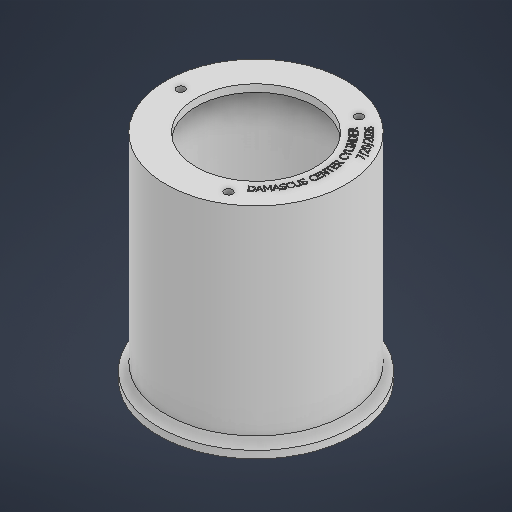
# Autodesk Inventor part: Mithril Center Cylinder
Saved by Autodesk Inventor 2026.3 (Build 303398000, 398)
## iProperties
Created: 2026-03-06
Part Number: Mithril Center Cylinder
Material: Generic
Document SubType Name: Modeling
Designer: mumin
Density: 1 g/cm^3
Appearance: Default
Author: mumin
Autodesk Inventor part; units mm, degrees
note: some values were not read from the file. Chosen so that the rebuilt part matches the saved one: direction of "Hole1".
ref_plane "YZ Plane" through (0, 0, 0) normal (1, 0, 0) x (0, 1, 0)
ref_plane "XZ Plane" through (0, 0, 0) normal (0, 1, 0) x (-1, 0, 0)
ref_plane "XY Plane" through (0, 0, 0) normal (0, 0, 1) x (1, 0, 0)
sketch "Sketch1" plane through (0, 0, 0) normal (1, 0, 0) x (0, 1, 0)
  line L0 (0, 0) -> (100, 0)
  line L1 (145, -40.5) -> (140, -40.5)
  line L2 (140, -40.5) -> (140, -56)
  line L3 (140, -56) -> (0, -56)
  line L4 (0, -56) -> (0, -66)
  line L5 (0, -66) -> (5, -66)
  line L6 (5, -66) -> (5, -61)
  line L7 (5, -61) -> (145, -61)
  line L8 (145, -61) -> (145, -40.5)
  line L9 (5, -66) -> (9.9531, -61)
  point P0 (142.5, -40.5)
  dimension "d0" = 100
  dimension "d1" = 81
  dimension "d2" = 122
  dimension "d3" = 145
  dimension "d4" = 5
  dimension "d5" = 5
  dimension "d6" = 5
  dimension "d7" = 10
  constraints: 20 end point, 7 perpendicular, 2 horizontal, 2 point on line, 1 midpoint
  measures "d0" distance of L0.start L0.end
  measures "d1" diameter of point (142.5, -40.5) L0
  measures "d2" diameter of L7 L0
  measures "d3" distance between parallel lines of L4 L8
  measures "d4" distance between parallel lines of L2 L8
  measures "d5" distance between parallel lines of L4 L6
  measures "d6" distance between parallel lines of L7 L3
  measures "d7" distance between parallel lines of L5 L3
revolve "Revolution1" add sketch "Sketch1" angle 360 about axis through (0, 0, 0) along (0, 1, 0)
sketch "Sketch2" plane through (0, 145, 0) normal (0, 1, 0) x (1, 0, 0)
  circle A0 centre (0, 0) radius 51
  point P0 (-51, 0)
  point P1 (25.5, -44.1673)
  point P2 (25.5, 44.1673)
  dimension "d9" = 102
  dimension "d12" = 360
  constraints: 1 coincident, 1 horizontal alignment, 6 other
hole "Hole1" at (-51, 145, 0) at (25.5, 145, 44.1673) at (25.5, 145, -44.1673) direction (0, -1, 0) diameter 5.5 end up to surface
sketch "Sketch3" plane through (0, 145, 0) normal (0, 1, 0) x (1, 0, 0)
  circle A0 centre (25.5, 44.1673) radius 2.75 projected
  circle A1 centre (25.5, -44.1673) radius 2.75 projected
  circle A2 centre (-51, 0) radius 2.75 projected
  circle A3 centre (0, 0) radius 40.5 projected
  circle A4 centre (0, 0) radius 61 projected
  spline S0 degree 2 poles (32.8898, -33.2836) (33.3048, -33.7392) (33.6033, -34.8089) (33.4798, -35.2962) knots 0 0 0 1 2 2 2
  spline S1 degree 2 poles (33.4798, -35.2962) (33.3713, -35.6861) (32.9491, -36.2679) (32.5447, -36.6362) knots 0 0 0 1 2 2 2
  line L0 (32.5447, -36.6362) -> (31.779, -37.3335)
  line L1 (31.779, -37.3335) -> (28.749, -34.0065)
  line L2 (28.749, -34.0065) -> (29.5066, -33.3165)
  spline S2 degree 2 poles (29.5066, -33.3165) (29.9757, -32.8893) (30.6373, -32.5433) (30.9389, -32.4954) knots 0 0 0 1 2 2 2
  spline S3 degree 2 poles (30.9389, -32.4954) (31.4537, -32.4162) (32.4478, -32.7983) (32.8898, -33.2836) knots 0 0 0 1 2 2 2
  spline S4 degree 2 poles (32.4238, -33.6981) (32.0752, -33.3152) (31.3282, -33.0041) (30.9375, -33.0788) knots 0 0 0 1 2 2 2
  spline S5 degree 2 poles (30.9375, -33.0788) (30.6638, -33.1357) (30.1761, -33.4072) (29.8769, -33.6797) knots 0 0 0 1 2 2 2
  line L3 (29.8769, -33.6797) -> (29.5398, -33.9867)
  line L4 (29.5398, -33.9867) -> (31.8725, -36.548)
  line L5 (31.8725, -36.548) -> (32.2095, -36.241)
  spline S6 degree 2 poles (32.2095, -36.241) (32.5034, -35.9734) (32.8623, -35.4739) (32.9276, -35.1827) knots 0 0 0 1 2 2 2
  spline S7 degree 2 poles (32.9276, -35.1827) (33.017, -34.8151) (32.7774, -34.0863) (32.4238, -33.6981) knots 0 0 0 1 2 2 2
  line L6 (34.5192, -34.8294) -> (32.2641, -30.6502)
  line L7 (32.2641, -30.6502) -> (32.7667, -30.1116)
  line L8 (32.7667, -30.1116) -> (37.0917, -32.0726)
  line L9 (37.0917, -32.0726) -> (36.6613, -32.5338)
  line L10 (36.6613, -32.5338) -> (35.4628, -31.9741)
  line L11 (35.4628, -31.9741) -> (34.291, -33.2299)
  line L12 (34.291, -33.2299) -> (34.9322, -34.3868)
  line L13 (34.9322, -34.3868) -> (34.5192, -34.8294)
  line L14 (34.9776, -31.7458) -> (32.9534, -30.8095)
  line L15 (32.9534, -30.8095) -> (34.0297, -32.7616)
  line L16 (34.0297, -32.7616) -> (34.9776, -31.7458)
  line L17 (39.7858, -28.6673) -> (39.4173, -29.1384)
  line L18 (39.4173, -29.1384) -> (36.3639, -26.7503)
  line L19 (36.3639, -26.7503) -> (37.7173, -29.2995)
  line L20 (37.7173, -29.2995) -> (37.4926, -29.5867)
  line L21 (37.4926, -29.5867) -> (34.6992, -28.8788)
  line L22 (34.6992, -28.8788) -> (37.7526, -31.2669)
  line L23 (37.7526, -31.2669) -> (37.4089, -31.7064)
  line L24 (37.4089, -31.7064) -> (33.8643, -28.9341)
  line L25 (33.8643, -28.9341) -> (34.3675, -28.2907)
  line L26 (34.3675, -28.2907) -> (37.0328, -28.9493)
  line L27 (37.0328, -28.9493) -> (35.7289, -26.55)
  line L28 (35.7289, -26.55) -> (36.2411, -25.895)
  line L29 (36.2411, -25.895) -> (39.7858, -28.6673)
  line L30 (40.0329, -28.3201) -> (37.0877, -24.595)
  line L31 (37.0877, -24.595) -> (37.4893, -23.9775)
  line L32 (37.4893, -23.9775) -> (42.0887, -25.1592)
  line L33 (42.0887, -25.1592) -> (41.7448, -25.688)
  line L34 (41.7448, -25.688) -> (40.4674, -25.3445)
  line L35 (40.4674, -25.3445) -> (39.531, -26.7844)
  line L36 (39.531, -26.7844) -> (40.363, -27.8127)
  line L37 (40.363, -27.8127) -> (40.0329, -28.3201)
  line L38 (39.95, -25.2037) -> (37.7941, -24.6325)
  line L39 (37.7941, -24.6325) -> (39.1925, -26.3684)
  line L40 (39.1925, -26.3684) -> (39.95, -25.2037)
  spline S8 degree 2 poles (42.9943, -23.6719) (42.7587, -24.1) (42.2493, -24.6022) (41.9756, -24.7971) knots 0 0 0 1 2 2 2
  line L41 (41.9756, -24.7971) -> (41.3174, -24.435)
  line L42 (41.3174, -24.435) -> (41.3385, -24.3966)
  spline S9 degree 2 poles (41.3385, -24.3966) (41.7237, -24.2714) (42.3525, -23.7641) (42.5195, -23.4606) knots 0 0 0 1 2 2 2
  spline S10 degree 2 poles (42.5195, -23.4606) (42.7586, -23.0261) (42.6419, -22.3834) (42.3448, -22.2199) knots 0 0 0 1 2 2 2
  spline S11 degree 2 poles (42.3448, -22.2199) (42.1084, -22.0898) (41.6861, -22.1613) (41.4737, -22.3732) knots 0 0 0 1 2 2 2
  spline S12 degree 2 poles (41.4737, -22.3732) (41.3224, -22.5272) (41.0851, -22.7921) (40.9028, -22.9873) knots 0 0 0 1 2 2 2
  spline S13 degree 2 poles (40.9028, -22.9873) (40.736, -23.1618) (40.3955, -23.3949) (40.1959, -23.4474) knots 0 0 0 1 2 2 2
  spline S14 degree 2 poles (40.1959, -23.4474) (39.9981, -23.4967) (39.5728, -23.4375) (39.3428, -23.311) knots 0 0 0 1 2 2 2
  spline S15 degree 2 poles (39.3428, -23.311) (38.8636, -23.0473) (38.6264, -21.9428) (38.9446, -21.3645) knots 0 0 0 1 2 2 2
  spline S16 degree 2 poles (38.9446, -21.3645) (39.1274, -21.0322) (39.5819, -20.5164) (39.8453, -20.3326) knots 0 0 0 1 2 2 2
  line L43 (39.8453, -20.3326) -> (40.4715, -20.6771)
  line L44 (40.4715, -20.6771) -> (40.4504, -20.7155)
  spline S17 degree 2 poles (40.4504, -20.7155) (40.1742, -20.8091) (39.5951, -21.2563) (39.4176, -21.579) knots 0 0 0 1 2 2 2
  spline S18 degree 2 poles (39.4176, -21.579) (39.2172, -21.9432) (39.3111, -22.5818) (39.5891, -22.7347) knots 0 0 0 1 2 2 2
  spline S19 degree 2 poles (39.5891, -22.7347) (39.8383, -22.8719) (40.2814, -22.7702) (40.4856, -22.5579) knots 0 0 0 1 2 2 2
  spline S20 degree 2 poles (40.4856, -22.5579) (40.6217, -22.4164) (41.0022, -21.9972) (41.138, -21.8638) knots 0 0 0 1 2 2 2
  spline S21 degree 2 poles (41.138, -21.8638) (41.4859, -21.5266) (42.1949, -21.4256) (42.5624, -21.6278) knots 0 0 0 1 2 2 2
  spline S22 degree 2 poles (42.5624, -21.6278) (42.7956, -21.7561) (43.1392, -22.1908) (43.2025, -22.4462) knots 0 0 0 1 2 2 2
  spline S23 degree 2 poles (43.2025, -22.4462) (43.2713, -22.7297) (43.1929, -23.3109) (42.9943, -23.6719) knots 0 0 0 1 2 2 2
  spline S24 degree 2 poles (44.7609, -20.1361) (44.5784, -20.5338) (44.0014, -21.0836) (43.6204, -21.2058) knots 0 0 0 1 2 2 2
  spline S25 degree 2 poles (43.6204, -21.2058) (43.2427, -21.3294) (42.324, -21.2331) (41.8069, -20.996) knots 0 0 0 1 2 2 2
  spline S26 degree 2 poles (41.8069, -20.996) (41.2932, -20.7603) (40.6509, -20.1488) (40.4831, -19.771) knots 0 0 0 1 2 2 2
  spline S27 degree 2 poles (40.4831, -19.771) (40.3205, -19.3996) (40.3392, -18.5977) (40.5292, -18.1834) knots 0 0 0 1 2 2 2
  spline S28 degree 2 poles (40.5292, -18.1834) (40.6234, -17.9779) (40.8488, -17.6439) (40.9651, -17.5127) knots 0 0 0 1 2 2 2
  spline S29 degree 2 poles (40.9651, -17.5127) (41.069, -17.3999) (41.3178, -17.181) (41.4531, -17.0786) knots 0 0 0 1 2 2 2
  line L45 (41.4531, -17.0786) -> (42.1094, -17.3796)
  line L46 (42.1094, -17.3796) -> (42.0896, -17.4227)
  spline S30 degree 2 poles (42.0896, -17.4227) (41.9899, -17.4652) (41.7009, -17.6054) (41.5369, -17.7268) knots 0 0 0 1 2 2 2
  spline S31 degree 2 poles (41.5369, -17.7268) (41.3793, -17.8431) (41.1012, -18.1609) (40.9917, -18.3995) knots 0 0 0 1 2 2 2
  spline S32 degree 2 poles (40.9917, -18.3995) (40.8716, -18.6614) (40.8728, -19.2276) (40.9977, -19.4975) knots 0 0 0 1 2 2 2
  spline S33 degree 2 poles (40.9977, -19.4975) (41.1275, -19.7656) (41.6724, -20.2482) (42.0669, -20.4291) knots 0 0 0 1 2 2 2
  spline S34 degree 2 poles (42.0669, -20.4291) (42.4879, -20.6222) (43.1872, -20.6982) (43.4766, -20.6183) knots 0 0 0 1 2 2 2
  spline S35 degree 2 poles (43.4766, -20.6183) (43.7578, -20.5386) (44.1746, -20.1721) (44.2932, -19.9136) knots 0 0 0 1 2 2 2
  spline S36 degree 2 poles (44.2932, -19.9136) (44.4011, -19.6782) (44.4691, -19.2239) (44.4543, -19.0286) knots 0 0 0 1 2 2 2
  spline S37 degree 2 poles (44.4543, -19.0286) (44.4365, -18.8399) (44.3594, -18.5358) (44.3253, -18.4439) knots 0 0 0 1 2 2 2
  line L47 (44.3253, -18.4439) -> (44.3435, -18.4041)
  line L48 (44.3435, -18.4041) -> (44.9932, -18.7021)
  spline S38 degree 2 poles (44.9932, -18.7021) (44.9939, -18.8669) (45.0004, -19.1587) (44.976, -19.3521) knots 0 0 0 1 2 2 2
  spline S39 degree 2 poles (44.976, -19.3521) (44.9535, -19.5585) (44.8733, -19.8908) (44.7609, -20.1361) knots 0 0 0 1 2 2 2
  spline S40 degree 2 poles (46.1061, -16.868) (45.9695, -17.2413) (45.5714, -17.7247) (45.3048, -17.8485) knots 0 0 0 1 2 2 2
  spline S41 degree 2 poles (45.3048, -17.8485) (45.0041, -17.9909) (44.3213, -17.9469) (43.8692, -17.7815) knots 0 0 0 1 2 2 2
  line L49 (43.8692, -17.7815) -> (41.2322, -16.8169)
  line L50 (41.2322, -16.8169) -> (41.4377, -16.2552)
  line L51 (41.4377, -16.2552) -> (44.0747, -17.2199)
  spline S42 degree 2 poles (44.0747, -17.2199) (44.3692, -17.3276) (44.7941, -17.3976) (44.9938, -17.3503) knots 0 0 0 1 2 2 2
  spline S43 degree 2 poles (44.9938, -17.3503) (45.2064, -17.2999) (45.5239, -16.9734) (45.6266, -16.6926) knots 0 0 0 1 2 2 2
  spline S44 degree 2 poles (45.6266, -16.6926) (45.7231, -16.4289) (45.6988, -15.954) (45.5689, -15.7784) knots 0 0 0 1 2 2 2
  spline S45 degree 2 poles (45.5689, -15.7784) (45.4468, -15.6133) (45.0805, -15.3939) (44.7962, -15.2899) knots 0 0 0 1 2 2 2
  line L52 (44.7962, -15.2899) -> (42.1455, -14.3202)
  line L53 (42.1455, -14.3202) -> (42.3509, -13.7586)
  line L54 (42.3509, -13.7586) -> (44.988, -14.7232)
  spline S46 degree 2 poles (44.988, -14.7232) (45.4298, -14.8849) (45.9948, -15.2935) (46.1278, -15.5984) knots 0 0 0 1 2 2 2
  spline S47 degree 2 poles (46.1278, -15.5984) (46.2526, -15.8731) (46.2489, -16.4776) (46.1061, -16.868) knots 0 0 0 1 2 2 2
  spline S48 degree 2 poles (47.2439, -13.2996) (47.1117, -13.77) (46.7295, -14.3746) (46.5071, -14.6265) knots 0 0 0 1 2 2 2
  line L55 (46.5071, -14.6265) -> (45.7839, -14.4232)
  line L56 (45.7839, -14.4232) -> (45.7958, -14.381)
  spline S49 degree 2 poles (45.7958, -14.381) (46.1426, -14.1717) (46.6398, -13.535) (46.7336, -13.2015) knots 0 0 0 1 2 2 2
  spline S50 degree 2 poles (46.7336, -13.2015) (46.8679, -12.7241) (46.6084, -12.1245) (46.2819, -12.0327) knots 0 0 0 1 2 2 2
  spline S51 degree 2 poles (46.2819, -12.0327) (46.0222, -11.9597) (45.6271, -12.1251) (45.4684, -12.3797) knots 0 0 0 1 2 2 2
  spline S52 degree 2 poles (45.4684, -12.3797) (45.356, -12.564) (45.1849, -12.8758) (45.0517, -13.1073) knots 0 0 0 1 2 2 2
  spline S53 degree 2 poles (45.0517, -13.1073) (44.9288, -13.3152) (44.65, -13.6194) (44.4676, -13.7158) knots 0 0 0 1 2 2 2
  spline S54 degree 2 poles (44.4676, -13.7158) (44.2862, -13.8087) (43.8585, -13.8476) (43.6058, -13.7765) knots 0 0 0 1 2 2 2
  spline S55 degree 2 poles (43.6058, -13.7765) (43.0792, -13.6284) (42.5976, -12.6065) (42.7763, -11.9711) knots 0 0 0 1 2 2 2
  spline S56 degree 2 poles (42.7763, -11.9711) (42.879, -11.6061) (43.2045, -11.0006) (43.4195, -10.7618) knots 0 0 0 1 2 2 2
  line L57 (43.4195, -10.7618) -> (44.1075, -10.9553)
  line L58 (44.1075, -10.9553) -> (44.0957, -10.9974)
  spline S57 degree 2 poles (44.0957, -10.9974) (43.8478, -11.1512) (43.3854, -11.7182) (43.2856, -12.0727) knots 0 0 0 1 2 2 2
  spline S58 degree 2 poles (43.2856, -12.0727) (43.1731, -12.4729) (43.4095, -13.0735) (43.7149, -13.1594) knots 0 0 0 1 2 2 2
  spline S59 degree 2 poles (43.7149, -13.1594) (43.9887, -13.2364) (44.3972, -13.0369) (44.5479, -12.7838) knots 0 0 0 1 2 2 2
  spline S60 degree 2 poles (44.5479, -12.7838) (44.6484, -12.6151) (44.9238, -12.1205) (45.0258, -11.9598) knots 0 0 0 1 2 2 2
  spline S61 degree 2 poles (45.0258, -11.9598) (45.2881, -11.5525) (45.9558, -11.2932) (46.3595, -11.4068) knots 0 0 0 1 2 2 2
  spline S62 degree 2 poles (46.3595, -11.4068) (46.6158, -11.4788) (47.049, -11.8242) (47.1687, -12.0586) knots 0 0 0 1 2 2 2
  spline S63 degree 2 poles (47.1687, -12.0586) (47.3, -12.319) (47.3555, -12.9029) (47.2439, -13.2996) knots 0 0 0 1 2 2 2
  spline S64 degree 2 poles (48.4975, -7.5488) (48.4271, -7.9807) (48.0164, -8.6638) (47.6815, -8.8826) knots 0 0 0 1 2 2 2
  spline S65 degree 2 poles (47.6815, -8.8826) (47.3501, -9.1019) (46.4388, -9.2526) (45.8773, -9.161) knots 0 0 0 1 2 2 2
  spline S66 degree 2 poles (45.8773, -9.161) (45.3194, -9.0701) (44.538, -8.6507) (44.2761, -8.3309) knots 0 0 0 1 2 2 2
  spline S67 degree 2 poles (44.2761, -8.3309) (44.0208, -8.0159) (43.8262, -7.2378) (43.8996, -6.7879) knots 0 0 0 1 2 2 2
  spline S68 degree 2 poles (43.8996, -6.7879) (43.936, -6.5647) (44.0648, -6.183) (44.1421, -6.0256) knots 0 0 0 1 2 2 2
  spline S69 degree 2 poles (44.1421, -6.0256) (44.2124, -5.8893) (44.3943, -5.6123) (44.4975, -5.4776) knots 0 0 0 1 2 2 2
  line L59 (44.4975, -5.4776) -> (45.2102, -5.5939)
  line L60 (45.2102, -5.5939) -> (45.2025, -5.6407)
  spline S70 degree 2 poles (45.2025, -5.6407) (45.1176, -5.7081) (44.8762, -5.92) (44.7502, -6.0805) knots 0 0 0 1 2 2 2
  spline S71 degree 2 poles (44.7502, -6.0805) (44.6291, -6.2344) (44.4452, -6.6145) (44.4029, -6.8736) knots 0 0 0 1 2 2 2
  spline S72 degree 2 poles (44.4029, -6.8736) (44.3565, -7.158) (44.5077, -7.7036) (44.6997, -7.9308) knots 0 0 0 1 2 2 2
  spline S73 degree 2 poles (44.6997, -7.9308) (44.896, -8.1549) (45.5494, -8.4757) (45.9777, -8.5456) knots 0 0 0 1 2 2 2
  spline S74 degree 2 poles (45.9777, -8.5456) (46.4347, -8.6201) (47.1292, -8.508) (47.387, -8.3542) knots 0 0 0 1 2 2 2
  spline S75 degree 2 poles (47.387, -8.3542) (47.6371, -8.2029) (47.9418, -7.739) (47.9876, -7.4582) knots 0 0 0 1 2 2 2
  spline S76 degree 2 poles (47.9876, -7.4582) (48.0293, -7.2027) (47.9744, -6.7467) (47.9084, -6.5623) knots 0 0 0 1 2 2 2
  spline S77 degree 2 poles (47.9084, -6.5623) (47.8412, -6.385) (47.6862, -6.1122) (47.6289, -6.0327) knots 0 0 0 1 2 2 2
  line L61 (47.6289, -6.0327) -> (47.636, -5.9895)
  line L62 (47.636, -5.9895) -> (48.3414, -6.1045)
  spline S78 degree 2 poles (48.3414, -6.1045) (48.3857, -6.2632) (48.4694, -6.5429) (48.4971, -6.7359) knots 0 0 0 1 2 2 2
  spline S79 degree 2 poles (48.4971, -6.7359) (48.5302, -6.9408) (48.541, -7.2825) (48.4975, -7.5488) knots 0 0 0 1 2 2 2
  line L63 (48.696, -5.5984) -> (44.2135, -5.2014)
  line L64 (44.2135, -5.2014) -> (44.4619, -2.3971)
  line L65 (44.4619, -2.3971) -> (44.9922, -2.4441)
  line L66 (44.9922, -2.4441) -> (44.7966, -4.6526)
  line L67 (44.7966, -4.6526) -> (46.0244, -4.7614)
  line L68 (46.0244, -4.7614) -> (46.2068, -2.7018)
  line L69 (46.2068, -2.7018) -> (46.7372, -2.7488)
  line L70 (46.7372, -2.7488) -> (46.5547, -4.8084)
  line L71 (46.5547, -4.8084) -> (48.2184, -4.9557)
  line L72 (48.2184, -4.9557) -> (48.414, -2.7472)
  line L73 (48.414, -2.7472) -> (48.9444, -2.7942)
  line L74 (48.9444, -2.7942) -> (48.696, -5.5984)
  line L75 (49.0145, 1.0806) -> (49.0073, 0.4096)
  line L76 (49.0073, 0.4096) -> (45.1059, -1.5394)
  line L77 (45.1059, -1.5394) -> (48.9858, -1.5813)
  line L78 (48.9858, -1.5813) -> (48.9797, -2.1393)
  line L79 (48.9797, -2.1393) -> (44.48, -2.0906)
  line L80 (44.48, -2.0906) -> (44.4892, -1.241)
  line L81 (44.4892, -1.241) -> (48.0714, 0.5328)
  line L82 (48.0714, 0.5328) -> (44.5088, 0.5713)
  line L83 (44.5088, 0.5713) -> (44.5148, 1.1292)
  line L84 (44.5148, 1.1292) -> (49.0145, 1.0806)
  line L85 (48.9066, 3.0386) -> (44.9483, 2.7681)
  line L86 (44.9483, 2.7681) -> (45.0512, 1.2619)
  line L87 (45.0512, 1.2619) -> (44.52, 1.2256)
  line L88 (44.52, 1.2256) -> (44.2734, 4.8347)
  line L89 (44.2734, 4.8347) -> (44.8046, 4.871)
  line L90 (44.8046, 4.871) -> (44.9075, 3.3648)
  line L91 (44.9075, 3.3648) -> (48.8659, 3.6353)
  line L92 (48.8659, 3.6353) -> (48.9066, 3.0386)
  line L93 (48.6962, 5.5962) -> (44.2406, 4.9659)
  line L94 (44.2406, 4.9659) -> (43.8462, 7.7534)
  line L95 (43.8462, 7.7534) -> (44.3734, 7.8279)
  line L96 (44.3734, 7.8279) -> (44.684, 5.6326)
  line L97 (44.684, 5.6326) -> (45.9044, 5.8053)
  line L98 (45.9044, 5.8053) -> (45.6148, 7.8526)
  line L99 (45.6148, 7.8526) -> (46.1419, 7.9271)
  line L100 (46.1419, 7.9271) -> (46.4316, 5.8798)
  line L101 (46.4316, 5.8798) -> (48.0853, 6.1138)
  line L102 (48.0853, 6.1138) -> (47.7747, 8.3091)
  line L103 (47.7747, 8.3091) -> (48.3019, 8.3837)
  line L104 (48.3019, 8.3837) -> (48.6962, 5.5962)
  line L105 (47.4399, 12.4311) -> (47.6057, 11.6723)
  line L106 (47.6057, 11.6723) -> (46.16, 9.9007)
  line L107 (46.16, 9.9007) -> (46.3063, 9.2309)
  line L108 (46.3063, 9.2309) -> (48.0556, 9.6131)
  line L109 (48.0556, 9.6131) -> (48.1832, 9.0288)
  line L110 (48.1832, 9.0288) -> (43.7869, 8.0683)
  line L111 (43.7869, 8.0683) -> (43.5394, 9.2012)
  spline S80 degree 2 poles (43.5394, 9.2012) (43.4569, 9.5788) (43.4275, 10.1062) (43.5266, 10.3705) knots 0 0 0 1 2 2 2
  spline S81 degree 2 poles (43.5266, 10.3705) (43.6256, 10.6347) (44.0339, 11.0039) (44.3795, 11.0794) knots 0 0 0 1 2 2 2
  spline S82 degree 2 poles (44.3795, 11.0794) (44.8605, 11.1845) (45.6198, 10.8353) (45.8685, 10.4491) knots 0 0 0 1 2 2 2
  line L112 (45.8685, 10.4491) -> (47.4399, 12.4311)
  spline S83 degree 2 poles (44.5589, 10.4803) (44.3665, 10.4383) (44.1004, 10.2383) (44.0354, 10.0748) knots 0 0 0 1 2 2 2
  spline S84 degree 2 poles (44.0354, 10.0748) (43.9807, 9.9322) (43.9854, 9.586) (44.0383, 9.3438) knots 0 0 0 1 2 2 2
  line L113 (44.0383, 9.3438) -> (44.1652, 8.7631)
  line L114 (44.1652, 8.7631) -> (45.8182, 9.1243)
  line L115 (45.8182, 9.1243) -> (45.7062, 9.6373)
  spline S85 degree 2 poles (45.7062, 9.6373) (45.6509, 9.8902) (45.4739, 10.2733) (45.3046, 10.3819) knots 0 0 0 1 2 2 2
  spline S86 degree 2 poles (45.3046, 10.3819) (45.1554, 10.4837) (44.7869, 10.5301) (44.5589, 10.4803) knots 0 0 0 1 2 2 2
  spline S87 degree 2 poles (46.2906, 16.315) (46.433, 15.9013) (46.3947, 15.1051) (46.2033, 14.7538) knots 0 0 0 1 2 2 2
  spline S88 degree 2 poles (46.2033, 14.7538) (46.0153, 14.4037) (45.284, 13.8395) (44.7461, 13.6543) knots 0 0 0 1 2 2 2
  spline S89 degree 2 poles (44.7461, 13.6543) (44.2116, 13.4702) (43.3248, 13.4696) (42.9427, 13.6273) knots 0 0 0 1 2 2 2
  spline S90 degree 2 poles (42.9427, 13.6273) (42.5686, 13.7839) (42.0288, 14.3771) (41.8804, 14.8081) knots 0 0 0 1 2 2 2
  spline S91 degree 2 poles (41.8804, 14.8081) (41.8068, 15.0218) (41.7395, 15.4191) (41.7331, 15.5943) knots 0 0 0 1 2 2 2
  spline S92 degree 2 poles (41.7331, 15.5943) (41.7305, 15.7476) (41.7595, 16.0777) (41.7867, 16.2452) knots 0 0 0 1 2 2 2
  line L116 (41.7867, 16.2452) -> (42.4694, 16.4803)
  line L117 (42.4694, 16.4803) -> (42.4848, 16.4355)
  spline S93 degree 2 poles (42.4848, 16.4355) (42.442, 16.3359) (42.3296, 16.0349) (42.2947, 15.8339) knots 0 0 0 1 2 2 2
  spline S94 degree 2 poles (42.2947, 15.8339) (42.2609, 15.641) (42.2789, 15.2191) (42.3644, 14.9708) knots 0 0 0 1 2 2 2
  spline S95 degree 2 poles (42.3644, 14.9708) (42.4581, 14.6984) (42.8497, 14.2894) (43.1264, 14.1803) knots 0 0 0 1 2 2 2
  spline S96 degree 2 poles (43.1264, 14.1803) (43.4053, 14.0758) (44.1328, 14.1026) (44.5431, 14.2439) knots 0 0 0 1 2 2 2
  spline S97 degree 2 poles (44.5431, 14.2439) (44.981, 14.3946) (45.5395, 14.8222) (45.6938, 15.0798) knots 0 0 0 1 2 2 2
  spline S98 degree 2 poles (45.6938, 15.0798) (45.8424, 15.3315) (45.8912, 15.8844) (45.7986, 16.1533) knots 0 0 0 1 2 2 2
  spline S99 degree 2 poles (45.7986, 16.1533) (45.7143, 16.3981) (45.4499, 16.7738) (45.3045, 16.905) knots 0 0 0 1 2 2 2
  spline S100 degree 2 poles (45.3045, 16.905) (45.1614, 17.0293) (44.8957, 17.1962) (44.8076, 17.2391) knots 0 0 0 1 2 2 2
  line L118 (44.8076, 17.2391) -> (44.7934, 17.2805)
  line L119 (44.7934, 17.2805) -> (45.4692, 17.5132)
  spline S101 degree 2 poles (45.4692, 17.5132) (45.5834, 17.3944) (45.7895, 17.1877) (45.9052, 17.0308) knots 0 0 0 1 2 2 2
  spline S102 degree 2 poles (45.9052, 17.0308) (46.0314, 16.866) (46.2027, 16.5702) (46.2906, 16.315) knots 0 0 0 1 2 2 2
  line L120 (40.1647, 19.2416) -> (43.0705, 18.8373)
  line L121 (43.0705, 18.8373) -> (44.8992, 19.6248)
  line L122 (44.8992, 19.6248) -> (45.1358, 19.0755)
  line L123 (45.1358, 19.0755) -> (43.364, 18.3125)
  line L124 (43.364, 18.3125) -> (41.6041, 15.899)
  line L125 (41.6041, 15.899) -> (41.3416, 16.5086)
  line L126 (41.3416, 16.5086) -> (42.7002, 18.3602)
  line L127 (42.7002, 18.3602) -> (40.4157, 18.6588)
  line L128 (40.4157, 18.6588) -> (40.1647, 19.2416)
  line L129 (42.8748, 23.7713) -> (44.0676, 21.4528)
  line L130 (44.0676, 21.4528) -> (40.0661, 19.3942)
  line L131 (40.0661, 19.3942) -> (39.7925, 19.926)
  line L132 (39.7925, 19.926) -> (43.3205, 21.741)
  line L133 (43.3205, 21.741) -> (42.4013, 23.5278)
  line L134 (42.4013, 23.5278) -> (42.8748, 23.7713)
  line L135 (41.8356, 25.5253) -> (42.7169, 24.0214)
  line L136 (42.7169, 24.0214) -> (42.3205, 23.7891)
  line L137 (42.3205, 23.7891) -> (42.031, 24.2831)
  line L138 (42.031, 24.2831) -> (38.9414, 22.4725)
  line L139 (38.9414, 22.4725) -> (39.2309, 21.9785)
  line L140 (39.2309, 21.9785) -> (38.8345, 21.7462)
  line L141 (38.8345, 21.7462) -> (37.9531, 23.2501)
  line L142 (37.9531, 23.2501) -> (38.3496, 23.4824)
  line L143 (38.3496, 23.4824) -> (38.639, 22.9884)
  line L144 (38.639, 22.9884) -> (41.7286, 24.7991)
  line L145 (41.7286, 24.7991) -> (41.4391, 25.293)
  line L146 (41.4391, 25.293) -> (41.8356, 25.5253)
  line L147 (39.6545, 28.829) -> (40.031, 28.2736)
  line L148 (40.031, 28.2736) -> (37.9367, 24.4483)
  line L149 (37.9367, 24.4483) -> (41.1483, 26.6256)
  line L150 (41.1483, 26.6256) -> (41.4614, 26.1638)
  line L151 (41.4614, 26.1638) -> (37.7367, 23.6386)
  line L152 (37.7367, 23.6386) -> (37.2599, 24.3419)
  line L153 (37.2599, 24.3419) -> (39.1919, 27.8413)
  line L154 (39.1919, 27.8413) -> (36.2429, 25.842)
  line L155 (36.2429, 25.842) -> (35.9298, 26.3038)
  line L156 (35.9298, 26.3038) -> (39.6545, 28.829)
  spline S103 degree 2 poles (35.1342, 30.9051) (35.6131, 31.2929) (36.6984, 31.5289) (37.1777, 31.3774) knots 0 0 0 1 2 2 2
  spline S104 degree 2 poles (37.1777, 31.3774) (37.5606, 31.2465) (38.1169, 30.7913) (38.4612, 30.3662) knots 0 0 0 1 2 2 2
  line L157 (38.4612, 30.3662) -> (39.1129, 29.5614)
  line L158 (39.1129, 29.5614) -> (35.6159, 26.7293)
  line L159 (35.6159, 26.7293) -> (34.971, 27.5257)
  spline S105 degree 2 poles (34.971, 27.5257) (34.5717, 28.0188) (34.2646, 28.6992) (34.2343, 29.0032) knots 0 0 0 1 2 2 2
  spline S106 degree 2 poles (34.2343, 29.0032) (34.1851, 29.5217) (34.6241, 30.492) (35.1342, 30.9051) knots 0 0 0 1 2 2 2
  spline S107 degree 2 poles (35.521, 30.4159) (35.1186, 30.09) (34.7647, 29.3623) (34.8166, 28.9679) knots 0 0 0 1 2 2 2
  spline S108 degree 2 poles (34.8166, 28.9679) (34.8575, 28.6914) (35.1003, 28.1888) (35.355, 27.8742) knots 0 0 0 1 2 2 2
  line L160 (35.355, 27.8742) -> (35.6419, 27.52)
  line L161 (35.6419, 27.52) -> (38.3341, 29.7003)
  line L162 (38.3341, 29.7003) -> (38.0473, 30.0545)
  spline S109 degree 2 poles (38.0473, 30.0545) (37.7971, 30.3634) (37.3192, 30.7507) (37.0323, 30.8327) knots 0 0 0 1 2 2 2
  spline S110 degree 2 poles (37.0323, 30.8327) (36.6705, 30.9433) (35.9291, 30.7464) (35.521, 30.4159) knots 0 0 0 1 2 2 2
  line L163 (36.4339, 32.7903) -> (33.1689, 29.6937)
  line L164 (33.1689, 29.6937) -> (31.2316, 31.7364)
  line L165 (31.2316, 31.7364) -> (31.6179, 32.1027)
  line L166 (31.6179, 32.1027) -> (33.1436, 30.494)
  line L167 (33.1436, 30.494) -> (34.0379, 31.3422)
  line L168 (34.0379, 31.3422) -> (32.6151, 32.8424)
  line L169 (32.6151, 32.8424) -> (33.0014, 33.2088)
  line L170 (33.0014, 33.2088) -> (34.4242, 31.7086)
  line L171 (34.4242, 31.7086) -> (35.6361, 32.8579)
  line L172 (35.6361, 32.8579) -> (34.1103, 34.4666)
  line L173 (34.1103, 34.4666) -> (34.4966, 34.833)
  line L174 (34.4966, 34.833) -> (36.4339, 32.7903)
  line L175 (31.4479, 37.6312) -> (32.0229, 37.109)
  line L176 (32.0229, 37.109) -> (31.872, 34.8273)
  line L177 (31.872, 34.8273) -> (32.3795, 34.3664)
  line L178 (32.3795, 34.3664) -> (33.5833, 35.6919)
  line L179 (33.5833, 35.6919) -> (34.026, 35.2899)
  line L180 (34.026, 35.2899) -> (31.0007, 31.9586)
  line L181 (31.0007, 31.9586) -> (30.1422, 32.7382)
  spline S111 degree 2 poles (30.1422, 32.7382) (29.8561, 32.9981) (29.5264, 33.4107) (29.4539, 33.6835) knots 0 0 0 1 2 2 2
  spline S112 degree 2 poles (29.4539, 33.6835) (29.3814, 33.9562) (29.5001, 34.4937) (29.7379, 34.7556) knots 0 0 0 1 2 2 2
  spline S113 degree 2 poles (29.7379, 34.7556) (30.0689, 35.12) (30.8901, 35.2757) (31.3165, 35.1052) knots 0 0 0 1 2 2 2
  line L182 (31.3165, 35.1052) -> (31.4479, 37.6312)
  spline S114 degree 2 poles (30.2314, 34.3715) (30.099, 34.2257) (29.9981, 33.9085) (30.0399, 33.7375) knots 0 0 0 1 2 2 2
  spline S115 degree 2 poles (30.0399, 33.7375) (30.078, 33.5896) (30.2825, 33.3103) (30.4661, 33.1436) knots 0 0 0 1 2 2 2
  line L183 (30.4661, 33.1436) -> (30.9061, 32.744)
  line L184 (30.9061, 32.744) -> (32.0436, 33.9966)
  line L185 (32.0436, 33.9966) -> (31.6549, 34.3496)
  spline S116 degree 2 poles (31.6549, 34.3496) (31.4632, 34.5237) (31.0969, 34.7332) (30.896, 34.7236) knots 0 0 0 1 2 2 2
  spline S117 degree 2 poles (30.896, 34.7236) (30.7154, 34.72) (30.3883, 34.5442) (30.2314, 34.3715) knots 0 0 0 1 2 2 2
  line L186 (47.9613, 21.9173) -> (52.2432, 21.617)
  line L187 (52.2432, 21.617) -> (52.4937, 21.026)
  line L188 (52.4937, 21.026) -> (48.0347, 21.3702)
  line L189 (48.0347, 21.3702) -> (48.9411, 19.2314)
  line L190 (48.9411, 19.2314) -> (48.4542, 19.0251)
  line L191 (48.4542, 19.0251) -> (47.3401, 21.6541)
  line L192 (47.3401, 21.6541) -> (47.9613, 21.9173)
  line L193 (46.196, 23.5365) -> (52.0733, 24.4297)
  line L194 (52.0733, 24.4297) -> (52.2961, 23.9703)
  line L195 (52.2961, 23.9703) -> (46.422, 23.0705)
  line L196 (46.422, 23.0705) -> (46.196, 23.5365)
  line L197 (48.8691, 28.4645) -> (50.2054, 26.0323)
  line L198 (50.2054, 26.0323) -> (49.6461, 25.725)
  spline S118 degree 2 poles (49.6461, 25.725) (49.256, 25.8519) (48.5426, 26.0674) (48.1736, 26.1559) knots 0 0 0 1 2 2 2
  spline S119 degree 2 poles (48.1736, 26.1559) (47.4306, 26.3344) (46.6553, 26.3369) (46.3389, 26.1631) knots 0 0 0 1 2 2 2
  spline S120 degree 2 poles (46.3389, 26.1631) (46.1727, 26.0718) (45.9796, 25.8325) (45.9506, 25.696) knots 0 0 0 1 2 2 2
  spline S121 degree 2 poles (45.9506, 25.696) (45.9216, 25.5594) (45.9752, 25.2726) (46.056, 25.1256) knots 0 0 0 1 2 2 2
  spline S122 degree 2 poles (46.056, 25.1256) (46.1332, 24.9849) (46.3616, 24.7359) (46.4879, 24.6347) knots 0 0 0 1 2 2 2
  spline S123 degree 2 poles (46.4879, 24.6347) (46.5941, 24.5474) (46.8361, 24.4099) (46.916, 24.3706) knots 0 0 0 1 2 2 2
  line L199 (46.916, 24.3706) -> (46.9318, 24.3418)
  line L200 (46.9318, 24.3418) -> (46.3693, 24.0328)
  spline S124 degree 2 poles (46.3693, 24.0328) (46.1998, 24.1519) (45.7219, 24.6507) (45.5779, 24.9128) knots 0 0 0 1 2 2 2
  spline S125 degree 2 poles (45.5779, 24.9128) (45.2741, 25.4657) (45.5165, 26.4103) (46.0151, 26.6842) knots 0 0 0 1 2 2 2
  spline S126 degree 2 poles (46.0151, 26.6842) (46.2484, 26.8124) (46.6981, 26.918) (46.9169, 26.9134) knots 0 0 0 1 2 2 2
  spline S127 degree 2 poles (46.9169, 26.9134) (47.1422, 26.9124) (47.6338, 26.8204) (47.881, 26.7566) knots 0 0 0 1 2 2 2
  spline S128 degree 2 poles (47.881, 26.7566) (48.2897, 26.6565) (49.2067, 26.3657) (49.4762, 26.2766) knots 0 0 0 1 2 2 2
  line L201 (49.4762, 26.2766) -> (48.4121, 28.2134)
  line L202 (48.4121, 28.2134) -> (48.8691, 28.4645)
  spline S129 degree 2 poles (45.166, 30.1524) (46.1904, 30.7977) (47.5252, 30.8066) (47.9158, 30.1864) knots 0 0 0 1 2 2 2
  spline S130 degree 2 poles (47.9158, 30.1864) (48.3123, 29.557) (47.7054, 28.3515) (46.7026, 27.7199) knots 0 0 0 1 2 2 2
  spline S131 degree 2 poles (46.7026, 27.7199) (45.672, 27.0707) (44.3435, 27.0656) (43.9509, 27.6889) knots 0 0 0 1 2 2 2
  spline S132 degree 2 poles (43.9509, 27.6889) (43.5563, 28.3153) (44.1725, 29.5266) (45.166, 30.1524) knots 0 0 0 1 2 2 2
  spline S133 degree 2 poles (46.7382, 30.2291) (46.5034, 30.1846) (45.8844, 29.8809) (45.4926, 29.634) knots 0 0 0 1 2 2 2
  spline S134 degree 2 poles (45.4926, 29.634) (45.1007, 29.3872) (44.5626, 28.962) (44.4168, 28.7625) knots 0 0 0 1 2 2 2
  spline S135 degree 2 poles (44.4168, 28.7625) (44.271, 28.5629) (44.2395, 28.1681) (44.3736, 27.9552) knots 0 0 0 1 2 2 2
  spline S136 degree 2 poles (44.3736, 27.9552) (44.5077, 27.7423) (44.8813, 27.594) (45.1323, 27.6401) knots 0 0 0 1 2 2 2
  spline S137 degree 2 poles (45.1323, 27.6401) (45.3753, 27.6854) (46.0027, 28.0031) (46.3761, 28.2382) knots 0 0 0 1 2 2 2
  spline S138 degree 2 poles (46.3761, 28.2382) (46.7772, 28.4909) (47.283, 28.8785) (47.4423, 29.0908) knots 0 0 0 1 2 2 2
  spline S139 degree 2 poles (47.4423, 29.0908) (47.5931, 29.2893) (47.633, 29.698) (47.4931, 29.9202) knots 0 0 0 1 2 2 2
  spline S140 degree 2 poles (47.4931, 29.9202) (47.3609, 30.13) (46.9874, 30.2783) (46.7382, 30.2291) knots 0 0 0 1 2 2 2
  line L203 (41.8171, 30.649) -> (47.4747, 32.4744)
  line L204 (47.4747, 32.4744) -> (47.7684, 32.0568)
  line L205 (47.7684, 32.0568) -> (42.115, 30.2255)
  line L206 (42.115, 30.2255) -> (41.8171, 30.649)
  line L207 (43.6642, 35.9424) -> (45.3738, 33.7563)
  line L208 (45.3738, 33.7563) -> (44.8711, 33.3632)
  spline S141 degree 2 poles (44.8711, 33.3632) (44.4657, 33.4258) (43.7269, 33.5239) (43.3485, 33.5521) knots 0 0 0 1 2 2 2
  spline S142 degree 2 poles (43.3485, 33.5521) (42.5865, 33.6089) (41.8208, 33.4869) (41.5364, 33.2645) knots 0 0 0 1 2 2 2
  spline S143 degree 2 poles (41.5364, 33.2645) (41.387, 33.1477) (41.2348, 32.8806) (41.2282, 32.7411) knots 0 0 0 1 2 2 2
  spline S144 degree 2 poles (41.2282, 32.7411) (41.2215, 32.6016) (41.3204, 32.3272) (41.4237, 32.195) knots 0 0 0 1 2 2 2
  spline S145 degree 2 poles (41.4237, 32.195) (41.5226, 32.0686) (41.788, 31.8595) (41.9289, 31.7799) knots 0 0 0 1 2 2 2
  spline S146 degree 2 poles (41.9289, 31.7799) (42.0477, 31.7108) (42.3087, 31.614) (42.3938, 31.588) knots 0 0 0 1 2 2 2
  line L209 (42.3938, 31.588) -> (42.414, 31.5621)
  line L210 (42.414, 31.5621) -> (41.9084, 31.1668)
  spline S147 degree 2 poles (41.9084, 31.1668) (41.7221, 31.2571) (41.1702, 31.6727) (40.986, 31.9083) knots 0 0 0 1 2 2 2
  spline S148 degree 2 poles (40.986, 31.9083) (40.5974, 32.4052) (40.685, 33.3765) (41.1331, 33.7269) knots 0 0 0 1 2 2 2
  spline S149 degree 2 poles (41.1331, 33.7269) (41.3428, 33.8909) (41.7697, 34.0673) (41.9864, 34.0979) knots 0 0 0 1 2 2 2
  spline S150 degree 2 poles (41.9864, 34.0979) (42.209, 34.1331) (42.7089, 34.1213) (42.9632, 34.098) knots 0 0 0 1 2 2 2
  spline S151 degree 2 poles (42.9632, 34.098) (43.3826, 34.0648) (44.3345, 33.925) (44.6148, 33.8803) knots 0 0 0 1 2 2 2
  line L211 (44.6148, 33.8803) -> (43.2534, 35.6211)
  line L212 (43.2534, 35.6211) -> (43.6642, 35.9424)
  spline S152 degree 2 poles (39.7381, 37.0138) (40.6456, 37.8152) (41.9616, 38.0383) (42.4468, 37.4889) knots 0 0 0 1 2 2 2
  spline S153 degree 2 poles (42.4468, 37.4889) (42.9392, 36.9313) (42.5338, 35.644) (41.6454, 34.8595) knots 0 0 0 1 2 2 2
  spline S154 degree 2 poles (41.6454, 34.8595) (40.7324, 34.0533) (39.4219, 33.835) (38.9343, 34.3871) knots 0 0 0 1 2 2 2
  spline S155 degree 2 poles (38.9343, 34.3871) (38.4443, 34.942) (38.858, 36.2365) (39.7381, 37.0138) knots 0 0 0 1 2 2 2
  spline S156 degree 2 poles (41.2777, 37.3419) (41.053, 37.2602) (40.4908, 36.8611) (40.1437, 36.5545) knots 0 0 0 1 2 2 2
  spline S157 degree 2 poles (40.1437, 36.5545) (39.7965, 36.248) (39.3337, 35.7419) (39.2218, 35.5215) knots 0 0 0 1 2 2 2
  spline S158 degree 2 poles (39.2218, 35.5215) (39.1099, 35.3011) (39.1423, 34.9064) (39.3088, 34.7178) knots 0 0 0 1 2 2 2
  spline S159 degree 2 poles (39.3088, 34.7178) (39.4754, 34.5292) (39.8679, 34.4428) (40.1083, 34.5287) knots 0 0 0 1 2 2 2
  spline S160 degree 2 poles (40.1083, 34.5287) (40.3409, 34.6124) (40.9091, 35.0266) (41.2399, 35.3187) knots 0 0 0 1 2 2 2
  spline S161 degree 2 poles (41.2399, 35.3187) (41.5952, 35.6325) (42.0322, 36.0963) (42.1553, 36.3315) knots 0 0 0 1 2 2 2
  spline S162 degree 2 poles (42.1553, 36.3315) (42.2723, 36.5516) (42.2461, 36.9614) (42.0723, 37.1582) knots 0 0 0 1 2 2 2
  spline S163 degree 2 poles (42.0723, 37.1582) (41.9082, 37.3441) (41.5157, 37.4304) (41.2777, 37.3419) knots 0 0 0 1 2 2 2
  line L213 (39.0712, 40.8884) -> (41.029, 38.9216)
  line L214 (41.029, 38.9216) -> (40.5767, 38.4714)
  spline S164 degree 2 poles (40.5767, 38.4714) (40.1667, 38.4852) (39.4215, 38.4947) (39.0425, 38.4775) knots 0 0 0 1 2 2 2
  spline S165 degree 2 poles (39.0425, 38.4775) (38.2791, 38.4431) (37.5334, 38.2308) (37.2775, 37.9761) knots 0 0 0 1 2 2 2
  spline S166 degree 2 poles (37.2775, 37.9761) (37.1431, 37.8423) (37.0239, 37.559) (37.0339, 37.4197) knots 0 0 0 1 2 2 2
  spline S167 degree 2 poles (37.0339, 37.4197) (37.0439, 37.2804) (37.1748, 37.0197) (37.2931, 36.9008) knots 0 0 0 1 2 2 2
  spline S168 degree 2 poles (37.2931, 36.9008) (37.4063, 36.7871) (37.6947, 36.6111) (37.8441, 36.5489) knots 0 0 0 1 2 2 2
  spline S169 degree 2 poles (37.8441, 36.5489) (37.9704, 36.4944) (38.241, 36.4293) (38.3286, 36.4137) knots 0 0 0 1 2 2 2
  line L215 (38.3286, 36.4137) -> (38.3517, 36.3904)
  line L216 (38.3517, 36.3904) -> (37.8969, 35.9376)
  spline S170 degree 2 poles (37.8969, 35.9376) (37.7011, 36.0051) (37.1036, 36.352) (36.8927, 36.5639) knots 0 0 0 1 2 2 2
  spline S171 degree 2 poles (36.8927, 36.5639) (36.4476, 37.0111) (36.4189, 37.9858) (36.8221, 38.3872) knots 0 0 0 1 2 2 2
  spline S172 degree 2 poles (36.8221, 38.3872) (37.0107, 38.575) (37.4135, 38.801) (37.6251, 38.8572) knots 0 0 0 1 2 2 2
  spline S173 degree 2 poles (37.6251, 38.8572) (37.8418, 38.9186) (38.3396, 38.9664) (38.5949, 38.9736) knots 0 0 0 1 2 2 2
  spline S174 degree 2 poles (38.5949, 38.9736) (39.0153, 38.9907) (39.977, 38.9653) (40.2606, 38.9543) knots 0 0 0 1 2 2 2
  line L217 (40.2606, 38.9543) -> (38.7016, 40.5205)
  line L218 (38.7016, 40.5205) -> (39.0712, 40.8884)
  spline S175 degree 2 poles (35.5393, 42.1043) (35.7698, 42.3629) (36.332, 42.6483) (36.6073, 42.6667) knots 0 0 0 1 2 2 2
  spline S176 degree 2 poles (36.6073, 42.6667) (36.8953, 42.6884) (37.4141, 42.5142) (37.6401, 42.3128) knots 0 0 0 1 2 2 2
  spline S177 degree 2 poles (37.6401, 42.3128) (37.866, 42.1114) (38.1031, 41.6266) (38.1088, 41.348) knots 0 0 0 1 2 2 2
  spline S178 degree 2 poles (38.1088, 41.348) (38.1204, 41.0103) (37.7705, 40.2231) (37.3726, 39.7766) knots 0 0 0 1 2 2 2
  spline S179 degree 2 poles (37.3726, 39.7766) (36.9819, 39.3383) (36.1738, 38.7934) (35.7531, 38.6994) knots 0 0 0 1 2 2 2
  spline S180 degree 2 poles (35.7531, 38.6994) (35.3426, 38.6061) (34.5107, 38.8347) (34.1323, 39.1719) knots 0 0 0 1 2 2 2
  spline S181 degree 2 poles (34.1323, 39.1719) (34.0207, 39.2714) (33.8441, 39.4679) (33.7924, 39.5579) knots 0 0 0 1 2 2 2
  line L219 (33.7924, 39.5579) -> (34.1782, 39.9908)
  line L220 (34.1782, 39.9908) -> (34.1973, 39.9738)
  spline S182 degree 2 poles (34.1973, 39.9738) (34.2308, 39.8853) (34.4085, 39.6243) (34.5392, 39.5078) knots 0 0 0 1 2 2 2
  spline S183 degree 2 poles (34.5392, 39.5078) (34.9584, 39.1342) (35.9776, 39.2418) (36.5216, 39.7535) knots 0 0 0 1 2 2 2
  spline S184 degree 2 poles (36.5216, 39.7535) (36.2615, 39.7851) (35.8147, 39.9634) (35.6133, 40.143) knots 0 0 0 1 2 2 2
  spline S185 degree 2 poles (35.6133, 40.143) (35.4173, 40.3177) (35.1936, 40.6587) (35.1398, 40.9216) knots 0 0 0 1 2 2 2
  spline S186 degree 2 poles (35.1398, 40.9216) (35.0784, 41.2254) (35.2821, 41.8157) (35.5393, 42.1043) knots 0 0 0 1 2 2 2
  spline S187 degree 2 poles (36.0136, 41.7157) (35.8292, 41.5088) (35.6882, 41.1313) (35.7206, 40.9266) knots 0 0 0 1 2 2 2
  spline S188 degree 2 poles (35.7206, 40.9266) (35.7474, 40.7757) (35.9294, 40.5305) (36.0464, 40.4262) knots 0 0 0 1 2 2 2
  spline S189 degree 2 poles (36.0464, 40.4262) (36.2043, 40.2854) (36.586, 40.1162) (36.8103, 40.0775) knots 0 0 0 1 2 2 2
  spline S190 degree 2 poles (36.8103, 40.0775) (36.8567, 40.124) (36.9447, 40.2117) (37.0077, 40.2825) knots 0 0 0 1 2 2 2
  spline S191 degree 2 poles (37.0077, 40.2825) (37.3183, 40.631) (37.5631, 41.1797) (37.5592, 41.3835) knots 0 0 0 1 2 2 2
  spline S192 degree 2 poles (37.5592, 41.3835) (37.5585, 41.5746) (37.4269, 41.8434) (37.3098, 41.9477) knots 0 0 0 1 2 2 2
  spline S193 degree 2 poles (37.3098, 41.9477) (37.0376, 42.1904) (36.3582, 42.1023) (36.0136, 41.7157) knots 0 0 0 1 2 2 2
  constraints: 1 other
emboss "Emboss1" sketch "Sketch3" operation cut depth 1 direction (0, -1, 0) contours S0 S1 L0 L1 L2 S2 S3 | L6 L7 L8 L9 L10 L11 L12 L13 | L17 L18 L19 L20 L21 L22 L23 L24 L25 L26 L27 L28 L29 | L30 L31 L32 L33 L34 L35 L36 L37 | S8 L41 L42 S9 S10 S11 S12 S13 S14 S15 S16 L43 L44 S17 S18 S19 S20 S21 S22 S23 | S24 S25 S26 S27 S28 S29 L45 L46 S30 S31 S32 S33 S34 S35 S36 S37 L47 L48 S38 S39 | S40 S41 L49 L50 L51 S42 S43 S44 S45 L52 L53 L54 S46 S47 | S48 L55 L56 S49 S50 S51 S52 S53 S54 S55 S56 L57 L58 S57 S58 S59 S60 S61 S62 S63 | S64 S65 S66 S67 S68 S69 L59 L60 S70 S71 S72 S73 S74 S75 S76 S77 L61 L62 S78 S79 | L63 L64 L65 L66 L67 L68 L69 L70 L71 L72 L73 L74 | L75 L76 L77 L78 L79 L80 L81 L82 L83 L84 | L85 L86 L87 L88 L89 L90 L91 L92 | L93 L94 L95 L96 L97 L98 L99 L100 L101 L102 L103 L104 | L105 L106 L107 L108 L109 L110 L111 S80 S81 S82 L112 | S87 S88 S89 S90 S91 S92 L124 L116 L117 S93 S94 S95 S96 S97 S98 S99 S100 L118 L119 S101 S102 | L124 L125 L126 L127 L128 L120 L121 L122 L123 L116 S92 | S92 L116 L124 | L129 L130 L131 L132 L133 L134 | L135 L136 L137 L138 L139 L140 L141 L142 L143 L144 L145 L146 | L147 L148 L149 L150 L151 L152 L153 L154 L155 L156 | S103 S104 L157 L158 L159 S105 S106 | L163 L164 L165 L166 L167 L168 L169 L170 L171 L172 L173 L174 | L175 L176 L177 L178 L179 L180 L181 S111 S112 S113 L182 | L186 L187 L188 L189 L190 L191 L192 | L193 L194 L195 L196 | L197 L198 S118 S119 S120 S121 S122 S123 L199 L200 S124 S125 S126 S127 S128 L201 L202 | S129 S130 S131 S132 | L203 L204 L205 L206 | L207 L208 S141 S142 S143 S144 S145 S146 L209 L210 S147 S148 S149 S150 S151 L211 L212 | S152 S153 S154 S155 | L213 L214 S164 S165 S166 S167 S168 S169 L215 L216 S170 S171 S172 S173 S174 L217 L218 | S175 S176 S177 S178 S179 S180 S181 L219 L220 S182 S183 S184 S185 S186
body "Solid1"
